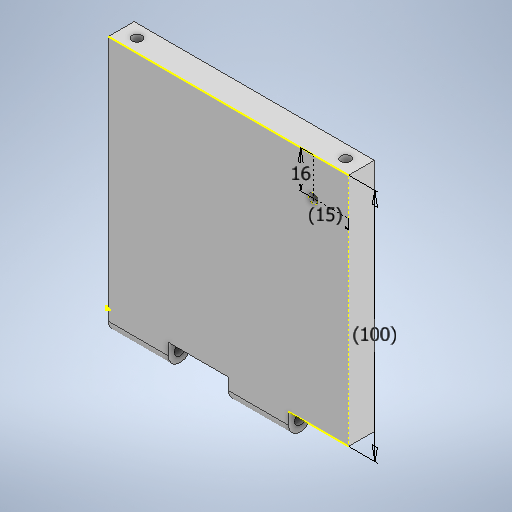
# Autodesk Inventor part: Hinge2
Saved by Autodesk Inventor 2025.1 (Build 291241000, 241)
## iProperties
Created: 2024-10-22
Part Number: Hinge2
Material: Generic
Document SubType Name: Modeling
Designer: vedan
Density: 1 g/cm^3
Appearance: Default
Author: vedan
Autodesk Inventor part; units mm, degrees
ref_plane "YZ Plane" through (0, 0, 0) normal (1, 0, 0) x (0, 1, 0)
ref_plane "XZ Plane" through (0, 0, 0) normal (0, 1, 0) x (-1, 0, 0)
ref_plane "XY Plane" through (0, 0, 0) normal (0, 0, 1) x (1, 0, 0)
sketch "Sketch1" plane through (0, 0, 0) normal (0, 0, 1) x (1, 0, 0)
  line L0 (0, 0) -> (102.3, 0)
  line L1 (102.3, 0) -> (102.3, 100)
  line L2 (102.3, 100) -> (0, 100)
  line L3 (0, 100) -> (0, 0)
  dimension "d0" = 102.3
  dimension "d1" = 100
  constraints: 8 end point, 2 parallel, 1 horizontal, 1 perpendicular
  measures "d0" distance of L2.end L1.end
  measures "d1" distance of L1.end L0.end
extrude "Extrusion1" add sketch "Sketch1" along normal blind 5
sketch "Sketch3" plane through (0, 0, 0) normal (-1, 0, 0) x (0, 0, 1)
  line L0 (5, 0) -> (0, 0)
  line L1 (0, 0) -> (0, -5)
  line L2 (0, -5) -> (5, -5)
  line L3 (5, -5) -> (5, 0)
  circle A0 centre (0, -5) radius 5
  circle A1 centre (0, -5) radius 2.5
  line L4 (-1.25, -2.8349) -> (-1.25, -0.1588)
  point P0 (0, 0)
  point P1 (0, -2.5)
  dimension "d15" = 5
  dimension "d16" = 5
  dimension "d17" = 5
  dimension "d18" = 2.5
  dimension "d19" = 1.25
  constraints: 10 end point, 2 parallel, 2 point on circle, 1 centre point, 1 coincident, 1 horizontal, 1 horizontal alignment, 1 perpendicular, 1 vertical, 1 vertical alignment, 3 other
  measures "d15" distance between parallel lines of L0 L2
  measures "d16" distance of L2.end L1.end
  measures "d17" distance of point (0, 0) L1.end
  measures "d19" distance between parallel lines of L1 L4
extrude "Extrusion3" add sketch "Sketch3" against normal blind 25.575 contours L3 A0 L0 | A0 L2 A1 L1 | A0 L4 A1 L2
pattern_linear "Rectangular Pattern2" count 2 spacing 51.15 along (1, 0, 0) of "Extrusion3"
sketch "Sketch4" plane through (0, 0, 0) normal (0, 0, -1) x (-1, 0, 0)
  point P0 (0, 0)
sketch "Sketch5" plane through (0, 0, 0) normal (0, 0, -1) x (-1, 0, 0)
  line L0 (-102.3, 0) -> (-102.3, 100) projected
  line L1 (0, 0) -> (-102.3, 0)
  line L2 (-102.3, 0) -> (-102.3, 100)
  line L3 (-102.3, 100) -> (0, 100)
  line L4 (0, 100) -> (0, 0)
  constraints: 8 end point, 2 parallel, 1 horizontal, 1 perpendicular
extrude "Extrusion4" add sketch "Sketch5" along normal blind 6
sketch "Sketch6" plane through (0, 0, 5) normal (0, 0, 1) x (1, 0, 0)
  line L0 (102.3, 100) -> (0, 100) construction
  line L1 (87.3, 100) -> (87.3, 84) construction
  line L2 (102.3, 0) -> (102.3, 100) construction
  point P0 (0, 0)
  dimension "d27" = 15
  dimension "d28" = 16
  constraints: 2 end point, 1 coincident, 1 perpendicular, 1 point on line
  measures "d27" distance between parallel lines of L1 L2
  measures "d28" distance of L1.start L1.end
hole "Hole1" at (87.3, 84, 5) direction (0, 0, -1) diameter 4 end through all
sketch "Sketch8" plane through (51.15, -5, 5) normal (-1, 0, 0) x (0, 0, 1)
  point P0 (-5, 5)
sketch "Sketch9" plane through (0, 0, 5) normal (0, 0, 1) x (1, 0, 0)
  circle A0 centre (87.3, 84) radius 2 construction
  line L0 (87.3, 84) -> (102.3, 84) construction
  line L1 (102.3, 0) -> (102.3, 100) construction
  line L2 (87.3, 84) -> (87.3, 100) construction
  line L3 (76.725, 0) -> (102.3, 0) projected
  line L4 (102.3, 100) -> (0, 100) projected
  point P0 (0, 0)
  dimension "d45" = 15
  dimension "d46" = 16
  dimension "d57" = 100
  constraints: 4 end point, 1 horizontal, 1 point on line, 1 vertical
  measures "d45" distance of L0.start L0.end
  measures "d46" distance of L0.start L2.end
  measures "d57" distance between parallel lines of L3 L4
sketch "Sketch10" plane through (0, 100, 5) normal (0, 1, 0) x (1, 0, 0)
  line L0 (0, 10) -> (0, 0) construction
  line L1 (0, 5.5) -> (102.7523, 5.5) construction
  line L2 (0, 11) -> (102.3, 11) construction
  point P0 (95.6, 5.5)
  point P1 (6.7, 5.5)
  point P2 (0, 6.25)
  dimension "d47" = 88.9
  dimension "d48" = 5.5
  dimension "d49" = 6.7
  constraints: 2 end point, 2 point on line, 1 horizontal
  measures "d47" distance of point (6.7, 5.5) point (95.6, 5.5)
  measures "d48" distance between parallel lines of L2 L1
  measures "d49" distance from line of L0 point (6.7, 5.5)
hole "Hole3" at (6.7, 100, -0.5) at (95.6, 100, -0.5) direction (0, -1, 0) diameter 4.25 depth 8 tip angle 118
body "Solid1"
